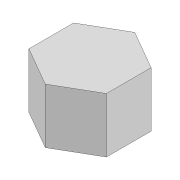
# Autodesk Inventor part: M4_lock_nut
Saved by Autodesk Inventor 2022 (Build 260153000, 153)
## iProperties
Created: 2022-08-15
Part Number: M4_lock_nut
Material: Generic
Document SubType Name: Modeling
Designer: dell
Density: 1 g/cm^3
Appearance: Default
Author: dell
Autodesk Inventor part; units mm, degrees
ref_plane "YZ Plane" through (0, 0, 0) normal (1, 0, 0) x (0, 1, 0)
ref_plane "XZ Plane" through (0, 0, 0) normal (0, 1, 0) x (-1, 0, 0)
ref_plane "XY Plane" through (0, 0, 0) normal (0, 0, 1) x (1, 0, 0)
sketch "Sketch1" plane through (0, 0, 0) normal (0, 1, 0) x (-1, 0, 0)
  line L0 (0, -3.9837) -> (-3.45, -1.9919)
  line L1 (-3.45, -1.9919) -> (-3.45, 1.9919)
  line L2 (-3.45, 1.9919) -> (0, 3.9837)
  line L3 (0, 3.9837) -> (3.45, 1.9919)
  line L4 (3.45, 1.9919) -> (3.45, -1.9919)
  line L5 (3.45, -1.9919) -> (0, -3.9837)
  point P0 (0, 0)
  point P1 (0, 0)
  dimension "d0" = 6.9
  constraints: 12 end point, 1 coincident, 13 other
  measures "d0" distance between parallel lines of L4 L1
extrude "Extrusion1" add sketch "Sketch1" along normal blind 4.9
body "Solid1"
